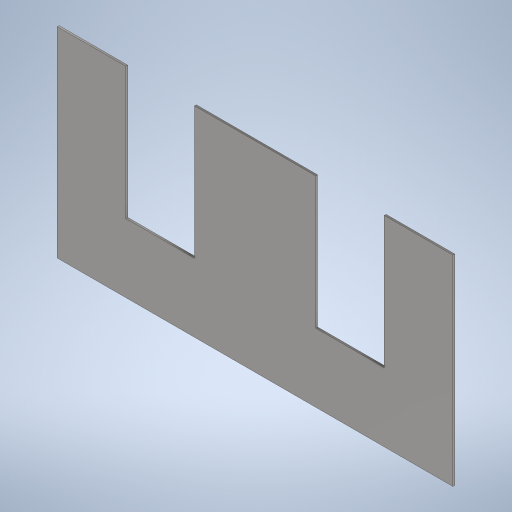
# Autodesk Inventor part: Chapa
Saved by Autodesk Inventor 2024.2 (Build 282272000, 272)
## iProperties
Created: 2024-05-06
Part Number: Chapa
Material: Steel, Alloy
Document SubType Name: Modeling
Designer: 082220019
Density: 7.73 g/cm^3
Appearance: Semi-Polished
Author: 082220019
Autodesk Inventor part; units mm, degrees
ref_plane "YZ Plane" through (0, 0, 0) normal (1, 0, 0) x (0, 1, 0)
ref_plane "XZ Plane" through (0, 0, 0) normal (0, 1, 0) x (-1, 0, 0)
ref_plane "XY Plane" through (0, 0, 0) normal (0, 0, 1) x (1, 0, 0)
sketch "Sketch1" plane through (0, 0, 0) normal (0, 0, 1) x (1, 0, 0)
  line L0 (0, 0) -> (0, 38)
  line L1 (0, 38) -> (13, 38)
  line L2 (13, 38) -> (13, 13)
  line L3 (13, 13) -> (26, 13)
  line L4 (26, 13) -> (26, 38)
  line L5 (26, 38) -> (49, 38)
  line L6 (49, 38) -> (49, 13)
  line L7 (49, 13) -> (62, 13)
  line L8 (62, 13) -> (62, 38)
  line L9 (62, 38) -> (75, 38)
  line L10 (75, 38) -> (75, 0)
  line L11 (75, 0) -> (0, 0)
  point P0 (19.5, 13)
  dimension "d0" = 23
  dimension "d1" = 13
  dimension "d2" = 13
  dimension "d3" = 38
  dimension "d4" = 75
  dimension "d5" = 13
  dimension "d6" = 13
  dimension "d7" = 13
  constraints: 24 end point, 6 point on line, 5 perpendicular, 2 parallel, 2 vertical, 1 collinear, 1 midpoint
  measures "d0" distance of L4.end L5.end
  measures "d1" distance of L0.end L1.end
  measures "d2" distance from line of L11 point (19.5, 13)
  measures "d3" distance of L9.end L10.end
  measures "d4" distance of L10.end L0.start
  measures "d5" distance of L4.end L1.end
  measures "d6" distance of L6.end L7.end
  measures "d7" distance of L8.end L9.end
extrude "Extrusion1" add sketch "Sketch1" along normal blind 0.3556
body "Solid1"
